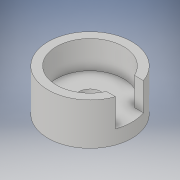
# Autodesk Inventor part: motor_mount
Saved by Autodesk Inventor 2019 (Build 230136000, 136)
## iProperties
Created: 2019-03-09
Part Number: motor_mount
Material: Generic
Document SubType Name: Modeling
Designer: Jaden
Density: 1 g/cm^3
Appearance: Default
Author: Jaden
Autodesk Inventor part; units mm, degrees
ref_plane "YZ Plane" through (0, 0, 0) normal (1, 0, 0) x (0, 1, 0)
ref_plane "XZ Plane" through (0, 0, 0) normal (0, 1, 0) x (-1, 0, 0)
ref_plane "XY Plane" through (0, 0, 0) normal (0, 0, 1) x (1, 0, 0)
sketch "Sketch1" plane through (0, 0, 0) normal (0, 1, 0) x (-1, 0, 0)
  circle A0 centre (0, 0) radius 12
  circle A1 centre (0, 0) radius 4
  circle A2 centre (0, 0) radius 15
  line L0 (-10.9087, -5) -> (-14.1421, -5)
  line L1 (-10.9087, 5) -> (-14.1421, 5)
  dimension "d0" = 5
  dimension "d2" = 10
  dimension "d3" = 8
  dimension "d4" = 30
  dimension "d5" = 3
  constraints: 4 end point, 4 point on circle, 3 centre point, 3 coincident, 2 horizontal
  measures "d0" distance from line of L0 point (0, 0)
  measures "d2" distance between parallel lines of L1 L0
  measures "d3" diameter of A1
  measures "d4" diameter of A2
  measures "d5" radial gap between concentric circles of A2 A0
extrude "Extrusion1" add sketch "Sketch1" along normal blind 15 contours A0 L1 A2 L0 picked at (13.8643, -1.1568)
sketch "Sketch2" plane through (0, 0, 0) normal (0, -1, 0) x (1, 0, 0)
  circle A0 centre (0, 0) radius 12
  circle A1 centre (0, 0) radius 4
  circle A2 centre (0, 0) radius 15
  line L0 (-10.9087, -5) -> (-14.1421, -5)
  line L1 (-10.9087, 5) -> (-14.1421, 5)
  dimension "d8" = 5
  dimension "d9" = 10
  dimension "d10" = 8
  dimension "d11" = 30
  dimension "d12" = 3
  constraints: 4 end point, 4 point on circle, 3 centre point, 3 coincident, 2 horizontal
  measures "d8" distance from line of L0 point (0, 0)
  measures "d9" distance between parallel lines of L1 L0
  measures "d10" diameter of A1
  measures "d11" diameter of A2
  measures "d12" radial gap between concentric circles of A2 A0
extrude "Extrusion2" add sketch "Sketch2" against normal blind 5 contours A0
sketch "Sketch3" plane through (0, 0, 0) normal (0, -1, 0) x (1, 0, 0)
  circle A0 centre (0, 0) radius 12
  circle A1 centre (0, 0) radius 4
  circle A2 centre (0, 0) radius 15
  line L0 (-10.9087, -5) -> (-14.1421, -5)
  line L1 (-10.9087, 5) -> (-14.1421, 5)
  dimension "d15" = 5
  dimension "d16" = 10
  dimension "d17" = 8
  dimension "d18" = 30
  dimension "d19" = 3
  constraints: 4 end point, 4 point on circle, 3 centre point, 3 coincident, 2 horizontal
  measures "d15" distance from line of L0 point (0, 0)
  measures "d16" distance between parallel lines of L1 L0
  measures "d17" diameter of A1
  measures "d18" diameter of A2
  measures "d19" radial gap between concentric circles of A2 A0
extrude "Extrusion3" add sketch "Sketch3" against normal blind 5 contours A0 L1 A2 L0 picked at (13.8643, -1.1568)
sketch "Sketch4" plane through (0, 0, 0) normal (0, -1, 0) x (1, 0, 0)
  circle A0 centre (0, 0) radius 12
  circle A1 centre (0, 0) radius 4
  circle A2 centre (0, 0) radius 15
  line L0 (-10.9087, -5) -> (-14.1421, -5)
  line L1 (-10.9087, 5) -> (-14.1421, 5)
  dimension "d22" = 5
  dimension "d23" = 10
  dimension "d24" = 8
  dimension "d25" = 30
  dimension "d26" = 3
  constraints: 4 end point, 4 point on circle, 3 centre point, 3 coincident, 2 horizontal
  measures "d22" distance from line of L0 point (0, 0)
  measures "d23" distance between parallel lines of L1 L0
  measures "d24" diameter of A1
  measures "d25" diameter of A2
  measures "d26" radial gap between concentric circles of A2 A0
extrude "Extrusion4" add sketch "Sketch4" against normal blind 2 contours A1
body "Solid1"
